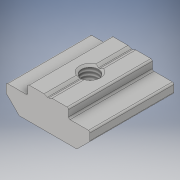
# Autodesk Inventor part: 13022_m
Saved by Autodesk Inventor 2019 (Build 230136000, 136)
## iProperties
Created: 2024-06-07
Part Number: 13022_m
Material: Generic
Catalog Web Link: www.cadenas.de
Description: 13022, 13023, 13024, 13025_m-Slide-In T-Nuts, Self-Aligning
Vendor: 8020
Document SubType Name: Modeling
Designer: psAdmin
Manufacturer: 8020
Mass: 1.14523 g
Surface Area: 8.34958 cm^2
Volume: 1.14523 cm^3
Density: 1 g/cm^3
Appearance: PSOLRGB-175-175-175
Category: PARTsolutions
Company: 8020
Title: 13022
Author: Cadenas PARTsolutions
Comments: Slide-In T-Nuts, Self-Aligning
PSOL_IDENT_0: {$CADENAS_DATA/23d-libs/8020/metric/fastening_options/13022_m.prj},175 {VTYP=3D},{NB=13022_m},{LINA=
PSOL_IDENT_1: 13022},{NN=13022, 13023, 13024, 13025_m},{DATE=27.07.2023 19:22:08},{GEOMDATE=24.06.2019 19:42:05},{
PSOL_IDENT_2: VERSION=},{LINEID=10},{WBVAR=A},{WBNUMERIC=}  {NB=13022_m},{LINA=13022},{KT=DUMMY},{PN=13022},{MAT=S
PSOL_IDENT_3: teel},{FIN=Zinc-Plated},{A=M4},{A1=4},{B=16.00},{C=16.00},{D=6.00},{E=7.80},{F=1.80},{W=.0840},{CC=8
PSOL_IDENT_4: -15, 8-30, 8-40},{R=0.30}
NB: 13022_m
NN: 13022, 13023, 13024, 13025_m
NT: Slide-In T-Nuts, Self-Aligning
NBSYN: $PN._m
LINA: 13022
CATALOG: 80/20
PN: 13022
MAT: Steel
FIN: Zinc-Plated
A: M4
B: 16
C: 16
D: 6
E: 7.8
F: 1.8
W: .0840
CC: 8-15, 8-30, 8-40
SUPPLIER: 8020
ARTICLENO: 13022_m
BOMINFO: 13022
CREATOR: CADENAS GmbH
Autodesk Inventor part; units mm, degrees
ref_plane "YZ Plane" through (0, 0, 0) normal (1, 0, 0) x (0, 1, 0)
ref_plane "XZ Plane" through (0, 0, 0) normal (0, 1, 0) x (-1, 0, 0)
ref_plane "XY Plane" through (0, 0, 0) normal (0, 0, 1) x (1, 0, 0)
sketch "Sketch_1" plane through (0, 0, 0) normal (0, 0, 1) x (1, 0, 0)
  arc A0 (-8, -1.5757) -> (-7.9121, -1.7879) centre (-7.7, -1.5757) ccw
  line L0 (-7.9121, -1.7879) -> (-5.5879, -4.1121)
  arc A1 (-5.5879, -4.1121) -> (-5.3757, -4.2) centre (-5.3757, -3.9) ccw
  line L1 (-5.3757, -4.2) -> (5.3757, -4.2)
  arc A2 (5.3757, -4.2) -> (5.5879, -4.1121) centre (5.3757, -3.9) ccw
  line L2 (5.5879, -4.1121) -> (7.9121, -1.7879)
  arc A3 (7.9121, -1.7879) -> (8, -1.5757) centre (7.7, -1.5757) ccw
  line L3 (8, -1.5757) -> (8, -0.3)
  arc A4 (8, -0.3) -> (7.7, 0) centre (7.7, -0.3) ccw
  line L4 (7.7, 0) -> (4.2, 0)
  arc A5 (3.9, 0.3) -> (4.2, 0) centre (4.2, 0.3) ccw
  line L5 (3.9, 0.3) -> (3.9, 1.5)
  arc A6 (3.9, 1.5) -> (3.6, 1.8) centre (3.6, 1.5) ccw
  line L6 (3.6, 1.8) -> (0.75, 1.8)
  line L7 (0.75, 1.8) -> (0.1124, 1.5424)
  arc A7 (-0.1124, 1.5424) -> (0.1124, 1.5424) centre (0, 1.8205) ccw
  line L8 (-0.1124, 1.5424) -> (-0.75, 1.8)
  line L9 (-0.75, 1.8) -> (-3.6, 1.8)
  arc A8 (-3.6, 1.8) -> (-3.9, 1.5) centre (-3.6, 1.5) ccw
  line L10 (-3.9, 1.5) -> (-3.9, 0.3)
  arc A9 (-4.2, 0) -> (-3.9, 0.3) centre (-4.2, 0.3) ccw
  line L11 (-4.2, 0) -> (-7.7, 0)
  arc A10 (-7.7, 0) -> (-8, -0.3) centre (-7.7, -0.3) ccw
  line L12 (-8, -0.3) -> (-8, -1.5757)
  constraints: 26 end point, 22 point on circle, 11 centre point
extrude "Extrusion1" add sketch "Sketch_1" along normal mid plane 16
sketch "Sketch_2" plane through (0, 0, 0) normal (1, 0, 0) x (0, 1, 0)
  line L0 (1.8, 0) -> (-4.2, 0)
  line L1 (-4.2, 0) -> (-4.2, 2)
  line L2 (-4.2, 2) -> (-3.821, 1.621)
  line L3 (-3.821, 1.621) -> (1.421, 1.621)
  line L4 (1.421, 1.621) -> (1.8, 2)
  line L5 (1.8, 2) -> (1.8, 0)
  line L6 (1.8, 0) -> (-4.2, 0)
  constraints: 14 end point
revolve "Revolution1" cut sketch "Sketch_2" angle 360 about axis through (0, 1.8, 0) along (0, 1, 0)
thread "Thread1" size "M4x0.7" class "6H" standard "ISO Metric profile" full length
body "Solid1"
